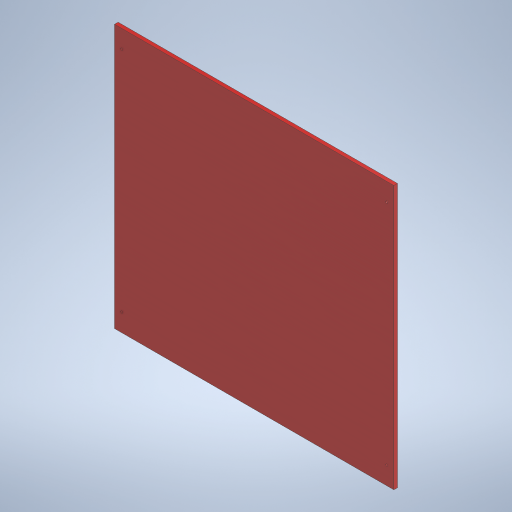
# Autodesk Inventor part: lamina
Saved by Autodesk Inventor 2023.2 (Build 272271030, 271C)
## iProperties
Created: 2023-03-05
Part Number: lamina
Material: Generic
Document SubType Name: Modeling
Designer: Cris Pat
Density: 1 g/cm^3
Appearance: Default
Author: Cris Pat
Autodesk Inventor part; units mm, degrees
ref_plane "YZ Plane" through (0, 0, 0) normal (1, 0, 0) x (0, 1, 0)
ref_plane "XZ Plane" through (0, 0, 0) normal (0, 1, 0) x (-1, 0, 0)
ref_plane "XY Plane" through (0, 0, 0) normal (0, 0, 1) x (1, 0, 0)
sketch "Sketch1" plane through (0, 0, 0) normal (0, 0, 1) x (1, 0, 0)
  line L0 (-390, 368) -> (390, 368)
  line L1 (390, 368) -> (390, -368)
  line L2 (390, -368) -> (-390, -368)
  line L3 (-390, -368) -> (-390, 368)
  line L4 (0, 368) -> (0, 0) construction
  line L5 (0, 0) -> (390, 0) construction
  circle A0 centre (370, 317.8995) radius 2.55
  circle A1 centre (-370, 317.8995) radius 2.55
  circle A2 centre (370, -317.8995) radius 2.55
  circle A3 centre (-370, -317.8995) radius 2.55
  point P0 (-390, 0)
  dimension "d0" = 736
  dimension "d1" = 780
  dimension "d2" = 5.1
  dimension "d3" = 317.8995
  dimension "d4" = 740
  constraints: 12 end point, 4 centre point, 3 midpoint, 3 symmetric about line, 2 parallel, 1 horizontal, 1 horizontal alignment, 1 perpendicular, 1 vertical, 1 vertical alignment, 3 other
  measures "d0" distance between parallel lines of L2 L0
  measures "d1" distance between parallel lines of L1 L3
  measures "d2" diameter of A0
  measures "d3" vertical distance of L5.end A0.centre
  measures "d4" distance of A1.centre A0.centre
extrude "Extrusion1" add sketch "Sketch1" along normal blind 10
body "Solid1"
